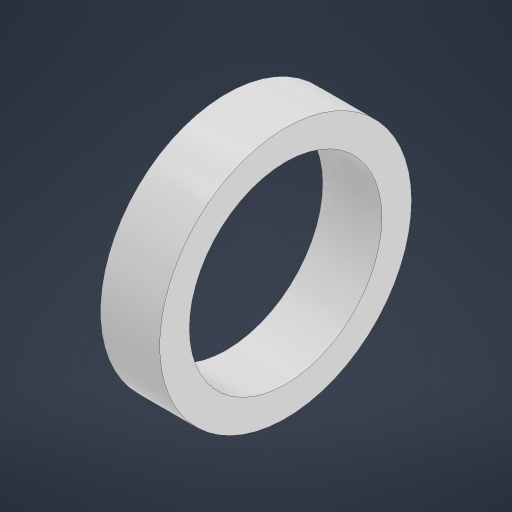
# Autodesk Inventor part: guide_profile
Saved by Autodesk Inventor 2024 (Build 280153000, 153)
## iProperties
Created: 2026-03-27
Part Number: guide_profile
Material: PET Plastic White
Document SubType Name: Modeling
Designer: schar
Density: 1.541 g/cm^3
Appearance: Polycarbonate - Clear(1)
Author: schar
Autodesk Inventor part; units mm, degrees
ref_plane "YZ Plane" through (0, 0, 0) normal (1, 0, 0) x (0, 1, 0)
ref_plane "XZ Plane" through (0, 0, 0) normal (0, 1, 0) x (-1, 0, 0)
ref_plane "XY Plane" through (0, 0, 0) normal (0, 0, 1) x (1, 0, 0)
sketch "Sketch1" plane through (0, 0, 0) normal (0, 1, 0) x (-1, 0, 0)
  circle A0 centre (0, 0) radius 2.8284
  line L0 (0, 0) -> (-2.8284, 0)
  line L1 (-2.8284, 0) -> (-2.8284, -2.8284)
  line L2 (-2.8284, -2.8284) -> (0, -2.8284)
  line L3 (0, -2.8284) -> (0, 0)
  line L4 (0, 0) -> (-2.8284, -2.8284)
  line L5 (2, 2) -> (-2, 2)
  line L6 (-2, 2) -> (-2, -2)
  line L7 (-2, -2) -> (2, -2)
  line L8 (2, -2) -> (2, 2)
  line L9 (2, 2) -> (-2, -2) construction
  line L10 (-2, 2) -> (2, -2) construction
  line L11 (2, 2) -> (-2, 2)
  line L12 (-2, 2) -> (-2, 4)
  line L13 (-2, 4) -> (2, 4)
  line L14 (2, 4) -> (2, 2)
  line L15 (0, 4) -> (0, 10.5)
  line L16 (2.8284, 10.5) -> (-3.1539, 10.5)
  dimension "d2" = 4
  dimension "d3" = 2
  dimension "d4" = 6.5
  dimension "d5" = 2
  constraints: 34 end point, 6 parallel, 5 horizontal, 3 midpoint, 3 perpendicular, 2 vertical, 1 coincident, 1 point on line, 3 other
  measures "d2" distance of L5.start L5.end
  measures "d3" distance of L11.end L12.end
  measures "d4" distance of L15.start L15.end
  measures "d5" distance between parallel lines of L15 L14
revolve "Revolution1" add sketch "Sketch1" angle 360 about axis through (-2.8284, 0, 10.5) along (1, 0, 0) contours L5 A0 | A0 L12 L13 L14
body "Solid1"
